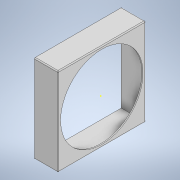
# Autodesk Inventor part: Base box
Saved by Autodesk Inventor 2020.2 (Build 242310000, 310)
## iProperties
Created: 2020-03-31
Part Number: Base box
Material: Generic
Document SubType Name: Modeling
Designer: Amaan Khalid
Density: 1 g/cm^3
Appearance: Default
Author: Amaan Khalid
Autodesk Inventor part; units mm, degrees
ref_plane "YZ Plane" through (0, 0, 0) normal (1, 0, 0) x (0, 1, 0)
ref_plane "XZ Plane" through (0, 0, 0) normal (0, 1, 0) x (-1, 0, 0)
ref_plane "XY Plane" through (0, 0, 0) normal (0, 0, 1) x (1, 0, 0)
sketch "Sketch1" plane through (0, 0, 0) normal (1, 0, 0) x (0, 1, 0)
  circle A0 centre (0, 0) radius 139.7
  line L0 (0, -139.7) -> (0, -146.05)
  line L1 (-139.7, 0) -> (-146.05, 0)
  line L2 (146.05, 0) -> (146.05, -146.05)
  line L3 (146.05, -146.05) -> (-146.05, -146.05)
  line L4 (-146.05, -146.05) -> (-146.05, 146.05)
  line L5 (-146.05, 146.05) -> (146.05, 146.05)
  line L6 (146.05, 146.05) -> (146.05, 0)
  dimension "d1" = 279.4
  constraints: 14 end point, 3 perpendicular, 2 horizontal, 2 point on circle, 2 vertical, 1 centre point, 1 coincident, 1 point on line
  measures "d1" diameter of A0
sketch "Sketch2" plane through (0, 0, 0) normal (0, 0, 1) x (1, 0, 0)
  point P0 (0, 0)
extrude "Extrusion1" add sketch "Sketch1" along normal blind 3.81 contours A0 L1 L4 L5 L6 L2 L3 L0 | A0 L0 L3 L4 L1
sketch "Sketch3" plane through (0, -146.05, 146.05) normal (0, 0, 1) x (1, 0, 0)
  line L0 (0, 292.1) -> (0, 0) projected
  line L1 (3.81, 292.1) -> (-76.2, 292.1)
  line L2 (-76.2, 292.1) -> (-76.2, 0)
  line L3 (-76.2, 0) -> (3.81, 0)
  point P0 (0, 146.05)
  dimension "d12" = 80.01
  constraints: 6 end point, 2 perpendicular, 1 horizontal
  measures "d12" distance of L1.start L1.end
extrude "Extrusion3" add sketch "Sketch3" along normal blind 2.54
sketch "Sketch4" plane through (3.81, -146.05, -146.05) normal (0, -1, 0) x (1, 0, 0)
  line L0 (-3.81, 292.1) -> (0, 292.1) projected
  line L1 (-3.81, 292.1) -> (-80.01, 292.1) projected
  line L2 (-3.81, 292.1) -> (-80.01, 292.1)
  line L3 (-3.81, 292.1) -> (-3.81, 0) projected
  line L4 (-3.81, 0) -> (-80.01, 0)
  line L5 (-80.01, 0) -> (-80.01, 292.1)
  point P0 (-3.81, 146.05)
  dimension "d15" = 76.2
  constraints: 6 end point, 1 collinear, 1 horizontal
  measures "d15" distance of L3.end L4.end
extrude "Extrusion4" add sketch "Sketch4" along normal blind 2.54
sketch "Sketch6" plane through (3.81, -146.05, -146.05) normal (0, 0, -1) x (-1, 0, 0)
  line L0 (80.01, 0) -> (3.81, 0) projected
  line L1 (3.81, 0) -> (80.01, 0)
  line L2 (80.01, 292.1) -> (80.01, 0) projected
  line L3 (80.01, 0) -> (80.01, 292.1)
  line L4 (80.01, 292.1) -> (3.81, 292.1)
  line L5 (3.81, 292.1) -> (3.81, 0)
  line L6 (3.81, 6.35) -> (3.81, 285.75) projected
  point P0 (3.81, 146.05)
  constraints: 8 end point, 2 perpendicular, 1 collinear, 1 horizontal
extrude "Extrusion5" add sketch "Sketch6" along normal blind 2.54
sketch "Sketch7" plane through (3.81, 146.05, 146.05) normal (0, 1, 0) x (1, 0, 0)
  line L0 (-3.81, 292.1) -> (0, 292.1) projected
  line L1 (-3.81, 292.1) -> (-80.01, 292.1)
  line L2 (-80.01, 292.1) -> (-80.01, 0)
  line L3 (-80.01, 0) -> (-3.81, 0)
  line L4 (-3.81, 292.1) -> (-3.81, 0)
  point P0 (-3.81, 146.05)
  constraints: 8 end point, 2 perpendicular, 1 horizontal, 1 vertical
extrude "Extrusion6" add sketch "Sketch7" along normal blind 2.54
sketch "Sketch21" plane through (-76.2, -148.59, -146.05) normal (-1, 0, 0) x (0, 0, 1)
  line L0 (0, 0) -> (-2.54, 0)
  line L1 (-2.54, 0) -> (-2.54, 2.54)
  line L2 (0, 2.54) -> (-2.54, 2.54) projected
  line L3 (-2.54, 2.54) -> (0, 2.54)
  line L4 (0, 2.54) -> (0, 0) projected
  line L5 (0, 2.54) -> (0, 0)
  point P0 (146.05, 148.59)
  constraints: 8 end point, 2 perpendicular, 1 collinear, 1 horizontal
extrude "Extrusion16" add sketch "Sketch21" against normal up to surface (76.2 mm away)
sketch "Sketch22" plane through (3.81, 148.59, 146.05) normal (0, 1, 0) x (1, 0, 0)
  line L0 (-3.81, 0) -> (-3.81, 294.64) projected
  line L1 (-80.01, 292.1) -> (-3.81, 292.1) projected
  line L2 (-3.81, 294.64) -> (-3.81, 292.1)
  line L3 (0, 292.1) -> (0, 0) projected
  line L4 (-3.81, 292.1) -> (0, 292.1)
  line L5 (0, 292.1) -> (0, 294.64)
  line L6 (0, 294.64) -> (-3.81, 294.64)
  point P0 (-3.81, 146.05)
  constraints: 8 end point, 4 perpendicular
extrude "Extrusion17" add sketch "Sketch22" against normal up to surface (297.18 mm away)
sketch "Sketch23" plane through (-76.2, -146.05, -146.05) normal (-1, 0, 0) x (0, 0, 1)
  line L0 (0, 292.1) -> (-2.54, 292.1) projected
  line L1 (-2.54, 292.1) -> (0, 292.1)
  line L2 (292.1, 294.64) -> (0, 294.64) projected
  line L3 (0, 292.1) -> (0, 294.64)
  line L4 (-2.54, 294.64) -> (-2.54, -2.54) projected
  line L5 (0, 294.64) -> (-2.54, 294.64)
  line L6 (-2.54, 294.64) -> (-2.54, 292.1)
  point P0 (146.05, 146.05)
  constraints: 8 end point, 2 perpendicular, 1 horizontal, 1 vertical
extrude "Extrusion18" add sketch "Sketch23" against normal up to surface (76.2 mm away)
sketch "Sketch26" plane through (0, -146.05, 148.59) normal (0, 0, 1) x (1, 0, 0)
  line L0 (0, 292.1) -> (3.81, 292.1) projected
  line L1 (3.81, 292.1) -> (0, 292.1)
  line L2 (0, 292.1) -> (0, 294.64) projected
  line L3 (0, 292.1) -> (0, 294.64)
  line L4 (0, 294.64) -> (3.81, 294.64)
  line L5 (3.81, 294.64) -> (3.81, 292.1)
  point P0 (0, 146.05)
  constraints: 8 end point, 2 collinear, 2 perpendicular
extrude "Extrusion20" add sketch "Sketch26" against normal up to surface (294.64 mm away)
sketch "Sketch27" plane through (0, -146.05, 148.59) normal (0, 0, 1) x (1, 0, 0)
  line L0 (0, 0) -> (3.81, 0) projected
  line L1 (3.81, 0) -> (0, 0)
  line L2 (0, 0) -> (0, -2.54) projected
  line L3 (0, 0) -> (0, -2.54)
  line L4 (0, -2.54) -> (3.81, -2.54) projected
  line L5 (0, -2.54) -> (3.81, -2.54)
  line L6 (3.81, 0) -> (3.81, -2.54) projected
  line L7 (3.81, -2.54) -> (3.81, 0)
  point P0 (0, 146.05)
  constraints: 8 end point, 2 collinear, 2 perpendicular
extrude "Extrusion21" add sketch "Sketch27" against normal up to surface (294.64 mm away)
sketch "Sketch28" plane through (0, 146.05, 148.59) normal (0, -1, 0) x (1, 0, 0)
  line L0 (3.81, 0) -> (3.81, -2.54) projected
  line L1 (3.81, 0) -> (3.81, -2.54)
  line L2 (3.81, -2.54) -> (0, -2.54)
  line L3 (0, -2.54) -> (0, 0)
  line L4 (0, 0) -> (3.81, 0)
  point P0 (0, -148.59)
  constraints: 8 end point, 3 perpendicular, 1 vertical
extrude "Extrusion22" add sketch "Sketch28" along normal up to surface (292.1 mm away)
sketch "Sketch29" plane through (-76.2, -146.05, -146.05) normal (-1, 0, 0) x (0, 0, 1)
  line L0 (292.1, 292.1) -> (294.64, 292.1) projected
  line L1 (294.64, 292.1) -> (292.1, 292.1)
  line L2 (292.1, 292.1) -> (292.1, 294.64) projected
  line L3 (292.1, 292.1) -> (292.1, 294.64)
  line L4 (294.64, 294.64) -> (294.64, 292.1) projected
  line L5 (292.1, 294.64) -> (294.64, 294.64)
  line L6 (294.64, 294.64) -> (294.64, 292.1)
  point P0 (146.05, 146.05)
  constraints: 8 end point, 3 perpendicular, 1 collinear
extrude "Extrusion23" add sketch "Sketch29" against normal up to surface (76.2 mm away)
sketch "Sketch30" plane through (-76.2, -146.05, -146.05) normal (-1, 0, 0) x (0, 0, 1)
  line L0 (292.1, 0) -> (0, 0) projected
  line L1 (292.1, 0) -> (292.1, -2.54)
  line L2 (294.64, -2.54) -> (-2.54, -2.54) projected
  line L3 (294.64, -2.54) -> (294.64, 0)
  line L4 (294.64, -2.54) -> (294.64, 294.64) projected
  line L5 (292.1, 0) -> (294.64, 0)
  line L6 (292.1, 0) -> (292.1, -2.54) projected
  line L7 (292.1, -2.54) -> (294.64, -2.54)
  point P0 (146.05, 146.05)
  constraints: 8 end point, 2 point on line, 1 parallel, 1 perpendicular, 1 vertical
extrude "Extrusion24" add sketch "Sketch30" against normal up to surface (76.2 mm away)
fillet "Fillet1" radius 3.175 8 edges at (-36.195, -148.59, 148.59) (-36.195, -148.59, -148.59) (-36.195, 148.59, -148.59) (-36.195, 148.59, 148.59) (3.81, 148.59, 0) (3.81, 0, 148.59) (3.81, 0, -148.59) (3.81, -148.59, 0)
body "Solid1"
